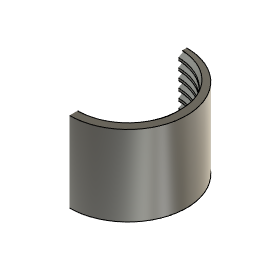
hilo (Autodesk Fusion 360 design; units mm, degrees)
Autodesk Fusion 360 part; units mm, degrees
sketch "Boceto1" plane through (0, 0, 0) normal (0, 0, 1) x (1, 0, 0)
  circle A0 centre (0, 0) radius 37.5
  circle A1 centre (0, 0) radius 40
  dimension "d1" = 75
  dimension "d2" = 80
  constraint coincident A0.centre A1.centre
  measures "d1" diameter of A0
  measures "d2" diameter of A1
extrude "Extruir3" add sketch "Boceto1" along normal blind 54.737 makes body 1
thread "Rosca3" "ISO Metric profile 75.0 M75x6 6H" major diameter 75.6205 minor diameter 68.9048 pitch 6 angle 60 modelled right hand crest width 1.6227 on face at (37.3137, -3.7338, 18.2457) crest through (34.4524, 0, 1.5) on bodies 1
sketch "Boceto3" plane through (0, 0, 0) normal (0, 0, 1) x (1, 0, 0)
  circle A0 centre (0, 0) radius 36.5
  dimension "d10" = 73
  constraint coincident A0.centre origin
  measures "d10" diameter of A0
extrude "Extruir4" add sketch "Boceto3" along normal blind 14.114 separate body makes body 2
thread "Rosca4" "ISO Metric profile 75.0 M75x6 6g" major diameter 74.62 minor diameter 67.7358 pitch 6 angle 60 modelled right hand crest width 0.8424 on face at (36.4546, -1.8194, 9.4093) crest through (37.31, 0, -1.5) on bodies 2
extrude "Extruir1" [rolled back] along distance 79.313 taper angle 0
thread "Rosca1" [rolled back]
sketch "Boceto2" plane through (0, 0, 0) normal (0, 0, 1) x (1, 0, 0)
  circle A0 centre (0, 0) radius 36.5
  dimension "d5" = 73
  constraint coincident A0.centre origin
  measures "d5" diameter of A0
extrude "Extruir2" [rolled back] along distance 25 taper angle 0
thread "Rosca2" [rolled back]
